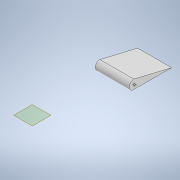
# Autodesk Inventor part: part
Saved by Autodesk Inventor 2021 (Build 250183000, 183)
## iProperties
Created: 2021-07-14
Part Number: part
Material: Generic
Document SubType Name: Modeling
Designer: Ashwin
Density: 1 g/cm^3
Appearance: Default
Author: Ashwin
Autodesk Inventor part; units mm, degrees
ref_plane "YZ Plane" through (0, 0, 0) normal (1, 0, 0) x (0, 1, 0)
ref_plane "XZ Plane" through (0, 0, 0) normal (0, 1, 0) x (-1, 0, 0)
ref_plane "XY Plane" through (0, 0, 0) normal (0, 0, 1) x (1, 0, 0)
sketch "Sketch1" plane through (0, 0, 0) normal (0, 1, 0) x (-1, 0, 0)
  line L0 (17.1429, -30) -> (-22.8571, -30)
  line L1 (-22.8571, -30) -> (-22.8571, -80)
  line L2 (-22.8571, -80) -> (17.1429, -80)
  line L3 (17.1429, -80) -> (17.1429, -30)
  point P0 (0, 0)
  dimension "d0" = 40
  dimension "d1" = 50
  constraints: 8 end point, 2 parallel, 1 horizontal, 1 perpendicular
  measures "d0" distance of L1.end L2.end
  measures "d1" distance of L0.end L1.end
extrude "Extrusion1" add sketch "Sketch1" along normal blind 10.475
sketch "Sketch3" plane through (22.8571, 0, -80) normal (0, 0, -1) x (-1, 0, 0)
  line L0 (0, 0) -> (40, 0) projected
  line L1 (0, 10.475) -> (40, 10.475)
  line L2 (40, 10.475) -> (40, 0)
  line L3 (40, 0) -> (0, 0)
  line L4 (0, 0) -> (0, 10.475)
  point P0 (22.8571, 0)
  constraints: 8 end point, 2 parallel, 1 horizontal, 1 perpendicular
extrude "Extrusion3" add sketch "Sketch3" along normal blind 11.252
full round fillet "Fillet1" first side at (9.5238, 10.475, -50.4173) centre faces at (9.5238, 3.4917, -91.252) second side at (9.5238, 0, -70.8347)
sketch "Sketch6" plane through (0, 0, 0) normal (0, -1, 0) x (1, 0, 0)
  line L0 (22.8571, -30) -> (22.8571, -86.0145) projected
  line L1 (-17.1429, -91.252) -> (-17.1429, -86.0145) projected
  line L2 (22.8571, -30) -> (-17.1429, -30)
  line L3 (-17.1429, -30) -> (-17.1429, -91.252)
  line L4 (-17.1429, -91.252) -> (22.8571, -91.252)
  line L5 (22.8571, -91.252) -> (22.8571, -30)
  point P0 (0, 0)
  constraints: 8 end point, 2 parallel, 1 horizontal, 1 perpendicular
extrude "Extrusion5" cut sketch "Sketch6" against normal blind 10.7
ref_plane "Work Plane5" through (0, 10.475, 0) normal (0, -1, 0) x (1, 0, 0)
sketch "Sketch8" plane through (0, 10.475, 0) normal (0, -1, 0) x (1, 0, 0)
  line L0 (-0.1429, -97) -> (-0.1429, -83) projected
  line L1 (-0.1429, -91.5044) -> (22.8571, -91.5044)
  line L2 (22.8571, -91.5044) -> (22.8571, -141.5044)
  line L3 (22.8571, -141.5044) -> (-0.1429, -141.5044)
  line L4 (-0.1429, -141.5044) -> (-0.1429, -91.5044)
  line L5 (-0.1429, -91.5044) -> (-17.1429, -91.5044)
  line L6 (-17.1429, -91.5044) -> (-17.1429, -141.5044)
  line L7 (-17.1429, -141.5044) -> (-0.1429, -141.5044)
  line L8 (-0.1429, -141.5044) -> (-0.1429, -91.5044)
  point P0 (0, 0)
  dimension "d14" = 23
  dimension "d15" = 50
  dimension "d16" = 17
  constraints: 16 end point, 4 parallel, 2 horizontal, 2 perpendicular, 1 point on line
  measures "d14" distance of L2.end L3.end
  measures "d15" distance of L3.end L1.start
  measures "d16" distance of L6.end L7.end
extrude "Extrusion6" add sketch "Sketch8" along normal blind 10.7
full round fillet "Fillet2" first side at (15.1905, 10.475, -124.8377) centre faces at (15.1905, 6.9083, -91.5044) second side at (15.1905, -0.225, -124.8377)
sketch "Sketch9" plane through (-17.1429, -0.225, -141.5044) normal (-1, 0, 0) x (0, 0, 1)
  line L0 (0, 10.7) -> (44.65, 10.7) projected
  line L1 (0, 10.7) -> (0, 0) projected
  line L2 (44.65, 10.7) -> (0, 0)
  line L3 (0, 0) -> (0, 10.7)
  arc A0 (44.65, 0) -> (44.65, 10.7) centre (44.65, 5.35) ccw projected
  line L4 (0, 10.7) -> (44.65, 10.7)
  point P0 (141.5044, 0.225)
  constraints: 6 end point, 1 collinear, 1 perpendicular, 1 tangent
extrude "Extrusion7" cut sketch "Sketch9" against normal blind 40
sketch "Sketch10" plane through (-17.1429, 5.125, -96.8544) normal (-1, 0, 0) x (0, 0, 1)
  line L0 (0, -1) -> (-0.866, -0.5)
  line L1 (-0.866, -0.5) -> (-0.866, 0.5)
  line L2 (-0.866, 0.5) -> (0, 1)
  line L3 (0, 1) -> (0.866, 0.5)
  line L4 (0.866, 0.5) -> (0.866, -0.5)
  line L5 (0.866, -0.5) -> (0, -1)
  point P0 (96.8544, -5.125)
  point P1 (0, 0)
  constraints: 12 end point, 13 other
extrude "Extrusion8" add sketch "Sketch10" along normal blind 2
sketch "Sketch11" plane through (22.8571, 5.125, -96.8544) normal (1, 0, 0) x (0, 0, -1)
  line L0 (0, -1) -> (-0.866, -0.5) projected
  line L1 (0, -1) -> (-0.866, -0.5)
  line L2 (-0.866, -0.5) -> (-0.866, 0.5)
  line L3 (-0.866, 0.5) -> (0, 1)
  line L4 (0, 1) -> (0.866, 0.5)
  line L5 (0.866, 0.5) -> (0.866, -0.5)
  line L6 (0.866, -0.5) -> (0, -1)
  point P0 (-96.8544, -5.125)
  point P1 (0, 0)
  constraints: 12 end point, 13 other
extrude "Extrusion9" add sketch "Sketch11" along normal blind 2
body "Solid1"
